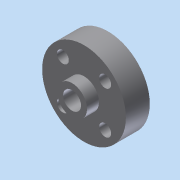
# Autodesk Inventor part: axle hub
Saved by Autodesk Inventor 2012 (Build 160160000, 160)
## iProperties
Created: 2011-10-31
Part Number: axle hub
Material: Default
Document SubType Name: Modeling
Designer: Kyle
Density: 1 g/cm^3
Author: Kyle
Autodesk Inventor part; units mm, degrees
ref_plane "YZ Plane" through (0, 0, 0) normal (1, 0, 0) x (0, 1, 0)
ref_plane "XZ Plane" through (0, 0, 0) normal (0, 1, 0) x (-1, 0, 0)
ref_plane "XY Plane" through (0, 0, 0) normal (0, 0, 1) x (1, 0, 0)
sketch "Sketch1" plane through (0, 0, 0) normal (0, 0, 1) x (1, 0, 0)
  circle A0 centre (0, 0) radius 11.1125
  circle A1 centre (0, 0) radius 2.3813
  circle A2 centre (0, 7.9375) radius 1.5875
  circle A3 centre (-7.9375, 0) radius 1.5875
  circle A4 centre (0, -7.9375) radius 1.5875
  circle A5 centre (7.9375, 0) radius 1.5875
  dimension "d0" = 22.225
  dimension "d1" = 4.7625
  dimension "d2" = 3.175
  dimension "d3" = 7.9375
  dimension "d6" = 360
  constraints: 6 centre point, 2 coincident, 9 other
  measures "d0" diameter of A0
  measures "d1" diameter of A1
  measures "d2" diameter of A2
  measures "d3" distance of A1.centre A2.centre
extrude "Extrusion1" add sketch "Sketch1" along normal blind 6.35
sketch "Sketch2" plane through (0, 0, 6.35) normal (0, 0, 1) x (1, 0, 0)
  circle A0 centre (0, 0) radius 2.3813 projected
  circle A1 centre (0, 0) radius 11.1125 projected
  circle A2 centre (0, 0) radius 3.9688
  circle A3 centre (0, 0) radius 2.3813
  dimension "d10" = 7.9375
  constraints: 2 centre point, 2 coincident, 1 concentric
  measures "d10" diameter of A2
extrude "Extrusion2" add sketch "Sketch2" along normal blind 3.175 contours A2
sketch "Sketch4" plane through (0, 0, 6.35) normal (0, 0, 1) x (1, 0, 0)
  circle A0 centre (0, 0) radius 3.9687 projected
  circle A1 centre (7.9375, 0) radius 1.5875 projected
  circle A2 centre (0, -7.9375) radius 1.5875 projected
  circle A3 centre (-7.9375, 0) radius 1.5875 projected
  circle A4 centre (0, 7.9375) radius 1.5875 projected
  circle A5 centre (0, 7.9375) radius 1.5875
  circle A6 centre (-7.9375, 0) radius 1.5875
  circle A7 centre (0, -7.9375) radius 1.5875
  circle A8 centre (7.9375, 0) radius 1.5875
  dimension "d22" = 360
  constraints: 4 centre point, 1 coincident, 1 concentric, 9 other
extrude "Extrusion3" add sketch "Sketch4" against normal blind 6.35 contours A1 | A2 | A3 | A4
sketch "Sketch5" plane through (0, 0, 6.35) normal (0, 0, 1) x (1, 0, 0)
  circle A0 centre (0, 0) radius 3.9687 projected
  circle A1 centre (0, 7.9375) radius 1.5875
  dimension "d26" = 3.175
  dimension "d27" = 7.9375
  constraints: 1 centre point
  measures "d26" diameter of A1
  measures "d27" distance of A0.centre A1.centre
hole "Hole2" at (0, 7.9375, 6.35) direction (0, 0, -1) diameter 3.175 end through all
pattern_circular "Circular Pattern1" count 8 over 360 about axis through (0, 0, 0) along (0, 0, 1) of "Hole2"
sketch "Sketch6" plane through (0, 0, 6.35) normal (0, 0, 1) x (1, 0, 0)
  circle A0 centre (7.9375, 0) radius 1.5875 projected
  circle A1 centre (0, -7.9375) radius 1.5875 projected
  circle A2 centre (-7.9375, 0) radius 1.5875 projected
  circle A3 centre (0, 7.9375) radius 1.5875 projected
  circle A4 centre (0, 0) radius 3.9687 projected
  circle A5 centre (0, 7.9375) radius 1.5875
  circle A6 centre (-7.9375, 0) radius 1.5875
  circle A7 centre (0, -7.9375) radius 1.5875
  circle A8 centre (7.9375, 0) radius 1.5875
  dimension "d40" = 360
  constraints: 4 centre point, 1 coincident, 1 concentric, 9 other
extrude "Extrusion4" add sketch "Sketch6" against normal blind 6.35 contours A0 | A1 | A2 | A3
body "Solid1"
